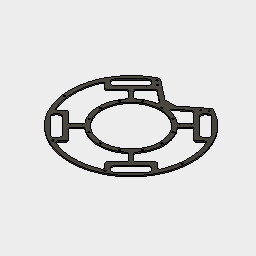
Bottom Plate (Autodesk Fusion 360 design; units mm, degrees)
Autodesk Fusion 360 part; units mm, degrees
sketch "Sketch1" plane through (0, 0, 0) normal (0, 1, 0) x (1, 0, 0)
  line L0 (69.2965, 69.2965) -> (82.7315, 55.8614)
  line L1 (82.7315, 47.3762) -> (80.6102, 45.2548)
  line L2 (72.1249, 45.2548) -> (45.2548, 72.1249)
  line L3 (45.2548, 80.6102) -> (47.3762, 82.7315)
  line L4 (55.8614, 82.7315) -> (69.2965, 69.2965)
  arc A0 (45.2548, 80.6102) -> (45.2548, 72.1249) centre (49.4975, 76.3675) ccw
  arc A1 (55.8614, 82.7315) -> (47.3762, 82.7315) centre (51.6188, 78.4889) ccw
  arc A2 (82.7315, 47.3762) -> (82.7315, 55.8614) centre (78.4889, 51.6188) ccw
  arc A3 (72.1249, 45.2548) -> (80.6102, 45.2548) centre (76.3675, 49.4975) ccw
  circle A4 centre (25.9155, 45.8559) radius 1.55
  circle A5 centre (45.8559, 25.9155) radius 1.55
  line L5 (-69.2965, 69.2965) -> (-55.8614, 82.7315)
  arc A6 (-45.2548, 72.1249) -> (-45.2548, 80.6102) centre (-49.4975, 76.3675) ccw
  circle A7 centre (-25.9155, 45.8559) radius 1.55
  line L6 (-82.7315, 55.8614) -> (-69.2965, 69.2965)
  arc A8 (-80.6102, 45.2548) -> (-72.1249, 45.2548) centre (-76.3675, 49.4975) ccw
  line L7 (-47.3762, 82.7315) -> (-45.2548, 80.6102)
  arc A9 (-47.3762, 82.7315) -> (-55.8614, 82.7315) centre (-51.6188, 78.4889) ccw
  arc A10 (-82.7315, 55.8614) -> (-82.7315, 47.3762) centre (-78.4889, 51.6188) ccw
  line L8 (-45.2548, 72.1249) -> (-72.1249, 45.2548)
  line L9 (-80.6102, 45.2548) -> (-82.7315, 47.3762)
  circle A11 centre (-45.8559, 25.9155) radius 1.55
  line L10 (-69.2965, -69.2965) -> (-82.7315, -55.8614)
  arc A12 (-72.1249, -45.2548) -> (-80.6102, -45.2548) centre (-76.3675, -49.4975) ccw
  circle A13 centre (-45.8559, -25.9155) radius 1.55
  line L11 (-55.8614, -82.7315) -> (-69.2965, -69.2965)
  arc A14 (-45.2548, -80.6102) -> (-45.2548, -72.1249) centre (-49.4975, -76.3675) ccw
  line L12 (-82.7315, -47.3762) -> (-80.6102, -45.2548)
  arc A15 (-82.7315, -47.3762) -> (-82.7315, -55.8614) centre (-78.4889, -51.6188) ccw
  arc A16 (-55.8614, -82.7315) -> (-47.3762, -82.7315) centre (-51.6188, -78.4889) ccw
  line L13 (-72.1249, -45.2548) -> (-45.2548, -72.1249)
  line L14 (-45.2548, -80.6102) -> (-47.3762, -82.7315)
  circle A17 centre (-25.9155, -45.8559) radius 1.55
  line L15 (69.2965, -69.2965) -> (55.8614, -82.7315)
  arc A18 (45.2548, -72.1249) -> (45.2548, -80.6102) centre (49.4975, -76.3675) ccw
  circle A19 centre (25.9155, -45.8559) radius 1.55
  line L16 (82.7315, -55.8614) -> (69.2965, -69.2965)
  arc A20 (80.6102, -45.2548) -> (72.1249, -45.2548) centre (76.3675, -49.4975) ccw
  line L17 (47.3762, -82.7315) -> (45.2548, -80.6102)
  arc A21 (47.3762, -82.7315) -> (55.8614, -82.7315) centre (51.6188, -78.4889) ccw
  arc A22 (82.7315, -55.8614) -> (82.7315, -47.3762) centre (78.4889, -51.6188) ccw
  line L18 (45.2548, -72.1249) -> (72.1249, -45.2548)
  line L19 (80.6102, -45.2548) -> (82.7315, -47.3762)
  circle A23 centre (45.8559, -25.9155) radius 1.55
  line L20 (-49.1439, -58.3363) -> (-33.234, -74.2462)
  line L21 (-58.3363, -49.1439) -> (-74.2462, -33.234)
  line L22 (-78.4889, -33.234) -> (-85.0774, -39.8226)
  line L23 (-39.8226, -85.0774) -> (-33.234, -78.4889)
  line L24 (49.1439, -58.3363) -> (33.234, -74.2462)
  line L25 (58.3363, -49.1439) -> (74.2462, -33.234)
  line L26 (85.0774, -39.8226) -> (78.4889, -33.234)
  line L27 (33.234, -78.4889) -> (39.8226, -85.0774)
  line L28 (58.3363, 49.1439) -> (74.2462, 33.234)
  line L29 (78.4889, 33.234) -> (85.0774, 39.8226)
  line L30 (-58.3363, 49.1439) -> (-74.2462, 33.234)
  line L31 (-85.0774, 39.8226) -> (-78.4889, 33.234)
  arc A24 (-38.8918, -89.9524) -> (38.8918, -89.9524) centre (0, 0) ccw
  arc A25 (89.9524, -38.8918) -> (89.9524, 38.8918) centre (0, 0) ccw
  arc A26 (-89.9524, 38.8918) -> (-89.9524, -38.8918) centre (0, 0) ccw
  arc A27 (-89.9524, -38.8918) -> (-85.0774, -39.8226) centre (-87.1987, -37.7012) ccw
  arc A28 (-74.2462, -33.234) -> (-78.4889, -33.234) centre (-76.3675, -35.3553) ccw
  arc A29 (-33.234, -78.4889) -> (-33.234, -74.2462) centre (-35.3553, -76.3675) ccw
  arc A30 (-39.8226, -85.0774) -> (-38.8918, -89.9524) centre (-37.7012, -87.1987) ccw
  arc A31 (38.8918, -89.9524) -> (39.8226, -85.0774) centre (37.7012, -87.1987) ccw
  arc A32 (33.234, -74.2462) -> (33.234, -78.4889) centre (35.3553, -76.3675) ccw
  arc A33 (78.4889, -33.234) -> (74.2462, -33.234) centre (76.3675, -35.3553) ccw
  arc A34 (85.0774, -39.8226) -> (89.9524, -38.8918) centre (87.1987, -37.7012) ccw
  arc A35 (89.9524, 38.8918) -> (85.0774, 39.8226) centre (87.1987, 37.7012) ccw
  arc A36 (74.2462, 33.234) -> (78.4889, 33.234) centre (76.3675, 35.3553) ccw
  arc A37 (-85.0774, 39.8226) -> (-89.9524, 38.8918) centre (-87.1987, 37.7012) ccw
  arc A38 (-78.4889, 33.234) -> (-74.2462, 33.234) centre (-76.3675, 35.3553) ccw
  circle A39 centre (0, 0) radius 49.1723
  line L32 (-49.1439, -54.0937) -> (-39.1131, -44.0628)
  line L33 (-54.0937, -49.1439) -> (-44.0628, -39.1131)
  line L34 (49.1439, -54.0937) -> (39.1131, -44.0628)
  line L35 (54.0937, -49.1439) -> (44.0628, -39.1131)
  line L36 (54.0937, 49.1439) -> (44.0628, 39.1131)
  line L37 (49.1439, 54.0937) -> (39.1131, 44.0628)
  line L38 (-54.0937, 49.1439) -> (-44.0628, 39.1131)
  line L39 (-49.1439, 54.0937) -> (-39.1131, 44.0628)
  arc A40 (43.8426, -35.1163) -> (43.8426, 35.1163) centre (0, 0) ccw
  arc A41 (-35.1163, -43.8426) -> (35.1163, -43.8426) centre (0, 0) ccw
  arc A42 (-43.8426, 35.1163) -> (-43.8426, -35.1163) centre (0, 0) ccw
  arc A43 (-39.1131, 44.0628) -> (-35.1163, 43.8426) centre (-36.9917, 46.1841) ccw
  arc A44 (-49.1439, 58.3363) -> (-49.1439, 54.0937) centre (-47.0226, 56.215) ccw
  arc A45 (-54.0937, 49.1439) -> (-58.3363, 49.1439) centre (-56.215, 47.0226) ccw
  arc A46 (-43.8426, 35.1163) -> (-44.0628, 39.1131) centre (-46.1841, 36.9917) ccw
  arc A47 (35.1163, 43.8426) -> (39.1131, 44.0628) centre (36.9917, 46.1841) ccw
  arc A48 (44.0628, 39.1131) -> (43.8426, 35.1163) centre (46.1841, 36.9917) ccw
  arc A49 (43.8426, -35.1163) -> (44.0628, -39.1131) centre (46.1841, -36.9917) ccw
  arc A50 (39.1131, -44.0628) -> (35.1163, -43.8426) centre (36.9917, -46.1841) ccw
  arc A51 (49.1439, -58.3363) -> (49.1439, -54.0937) centre (47.0226, -56.215) ccw
  arc A52 (58.3363, 49.1439) -> (54.0937, 49.1439) centre (56.215, 47.0226) ccw
  arc A53 (49.1439, 54.0937) -> (49.1439, 58.3363) centre (47.0226, 56.215) ccw
  arc A54 (-58.3363, -49.1439) -> (-54.0937, -49.1439) centre (-56.215, -47.0226) ccw
  arc A55 (-49.1439, -54.0937) -> (-49.1439, -58.3363) centre (-47.0226, -56.215) ccw
  arc A56 (-44.0628, -39.1131) -> (-43.8426, -35.1163) centre (-46.1841, -36.9917) ccw
  arc A57 (-35.1163, -43.8426) -> (-39.1131, -44.0628) centre (-36.9917, -46.1841) ccw
  arc A58 (54.0937, -49.1439) -> (58.3363, -49.1439) centre (56.215, -47.0226) ccw
  circle A59 centre (0, 52.6723) radius 1.55
  circle A60 centre (-52.6723, 0) radius 1.55
  circle A61 centre (0, -52.6723) radius 1.55
  circle A62 centre (52.6723, 0) radius 1.55
  circle A63 centre (44.8286, -89.3777) radius 1.55
  circle A64 centre (-44.8286, -89.3777) radius 1.55
  circle A65 centre (-44.8298, 89.3777) radius 1.55
  circle A66 centre (44.8298, 89.3777) radius 1.55
  line L40 (7.8776, 67) -> (-7.8776, 67)
  line L41 (43.2519, 93.8511) -> (9.7255, 67.6367)
  line L42 (-9.7255, 67.6367) -> (-43.2519, 93.8511)
  line L43 (-11.323, 60) -> (-11.3737, 60.0396)
  line L44 (49.1439, 58.3363) -> (33.4919, 73.9883)
  line L45 (29.5227, 74.2303) -> (11.3737, 60.0396)
  line L46 (-49.1439, 58.3363) -> (-33.4919, 73.9883)
  line L47 (-29.5227, 74.2303) -> (-11.323, 60)
  arc A67 (-12.5512, 54.7521) -> (-35.1163, 43.8426) centre (0, 0) ccw
  arc A68 (35.1163, 43.8426) -> (12.5512, 54.7521) centre (0, 0) ccw
  arc A69 (-29.5227, 74.2303) -> (-33.4919, 73.9883) centre (-31.3706, 71.867) ccw
  arc A70 (-12.5512, 54.7521) -> (-11.3737, 60.0396) centre (-13.2216, 57.6763) ccw
  arc A71 (11.3737, 60.0396) -> (12.5512, 54.7521) centre (13.2216, 57.6763) ccw
  arc A72 (33.4919, 73.9883) -> (29.5227, 74.2303) centre (31.3706, 71.867) ccw
  arc A73 (-43.2519, 93.8511) -> (-46.4263, 94.1785) centre (-45.0998, 91.4877) ccw
  arc A74 (-9.7255, 67.6367) -> (-7.8776, 67) centre (-7.8776, 70) ccw
  arc A75 (7.8776, 67) -> (9.7255, 67.6367) centre (7.8776, 70) ccw
  arc A76 (46.4263, 94.1785) -> (43.2519, 93.8511) centre (45.0998, 91.4877) ccw
  circle A77 centre (100.6317, -13.2484) radius 1.55
  circle A78 centre (-100.6317, -13.2484) radius 1.55
  arc A79 (-46.4263, 94.1785) -> (46.4263, 94.1785) centre (0, 0) ccw
  circle A80 centre (-37, 82.5) radius 1.5
  circle A81 centre (37, 82.5) radius 1.5
  point P0 (86.9741, 51.6188)
  point P1 (76.3675, 41.0122)
  point P2 (41.0122, 76.3675)
  point P3 (51.6188, 86.9741)
  point P4 (-86.9741, 51.6188)
  point P5 (-41.0122, 76.3675)
  point P6 (-51.6188, 86.9741)
  point P7 (-76.3675, 41.0122)
  point P8 (-51.6188, -86.9741)
  point P9 (-76.3675, -41.0122)
  point P10 (-86.9741, -51.6188)
  point P11 (-41.0122, -76.3675)
  point P12 (86.9741, -51.6188)
  point P13 (41.0122, -76.3675)
  point P14 (51.6188, -86.9741)
  point P15 (76.3675, -41.0122)
  point P16 (-31.1127, -76.3675)
  dimension "d176" = 3
  dimension "d177" = 3
  measures "d176" diameter of A81
  measures "d177" diameter of A80
extrude "Extrude1" add sketch "Sketch1" along normal blind 2
